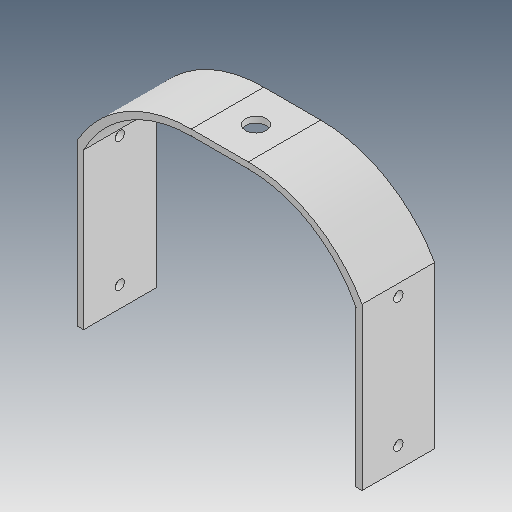
# Autodesk Inventor part: shin_bracket
Saved by Autodesk Inventor 2025.2 (Build 292293000, 293)
## iProperties
Created: 2025-02-16
Part Number: shin_bracket
Material: Generic
Document SubType Name: Modeling
Designer: email
Density: 1 g/cm^3
Appearance: Default
Author: email
Autodesk Inventor part; units mm, degrees
ref_plane "YZ Plane" through (0, 0, 0) normal (1, 0, 0) x (0, 1, 0)
ref_plane "XZ Plane" through (0, 0, 0) normal (0, 1, 0) x (-1, 0, 0)
ref_plane "XY Plane" through (0, 0, 0) normal (0, 0, 1) x (1, 0, 0)
sketch "Sketch1" plane through (0, 0, 0) normal (0, 0, 1) x (1, 0, 0)
  line L0 (0, 0) -> (3.2, 0)
  line L1 (3.2, 0) -> (3.2, 82)
  line L2 (0, 0) -> (0, 85)
  line L3 (146.8, 82) -> (146.8, 0)
  line L4 (146.8, 0) -> (150, 0)
  line L5 (150, 0) -> (150, 85)
  arc A0 (60, 116.8) -> (3.2, 82) centre (60, 53.046) ccw
  line L6 (60, 116.8) -> (90, 116.8)
  arc A1 (146.8, 82) -> (90, 116.8) centre (90, 53.046) ccw
  arc A2 (60, 120) -> (0, 85) centre (60, 51.0714) ccw
  line L7 (60, 120) -> (90, 120)
  arc A3 (150, 85) -> (90, 120) centre (90, 51.0714) ccw
  point P0 (75, 120)
  point P1 (75, 116.8)
  dimension "d0" = 3.2
  dimension "d1" = 3.2
  dimension "d2" = 3.2
  dimension "d3" = 150
  dimension "d4" = 120
  dimension "d5" = 30
  dimension "d12" = 85
  dimension "d13" = 75
  dimension "d14" = 3
  dimension "d15" = 30
  dimension "d16" = 85
  dimension "d17" = 8
  constraints: 16 end point, 8 point on circle, 4 centre point, 4 tangent, 3 perpendicular, 2 horizontal, 2 midpoint, 2 vertical, 1 collinear, 1 horizontal alignment, 1 parallel, 1 vertical alignment
  measures "d0" distance between parallel lines of L2 L1
  measures "d1" distance between parallel lines of L5 L3
  measures "d2" distance between parallel lines of L6 L7
  measures "d3" distance between parallel lines of L5 L2
  measures "d4" distance between parallel lines of L0 L7
  measures "d5" distance of L7.start L7.end
  measures "d12" distance of L4.end L5.end
  measures "d13" distance from line of L5 point (75, 120)
  measures "d14" vertical distance of L5.end L3.start
  measures "d15" distance of L6.start L6.end
  measures "d16" distance of L0.start L2.end
extrude "Extrusion1" add sketch "Sketch1" along normal blind 38.2
sketch "Sketch2" plane through (150, 0, 0) normal (1, 0, 0) x (0, 0, -1)
  circle A0 centre (-19.1, 11) radius 2.5
  circle A1 centre (-19.1, 79) radius 2.5
  line L0 (0, 0) -> (0, 85) projected
  line L1 (0, 0) -> (-38.2, 0) projected
  dimension "d8" = 19.1
  dimension "d9" = 5
  dimension "d10" = 68
  dimension "d11" = 11
  constraints: 2 centre point, 1 equal radius, 1 vertical alignment
  measures "d8" distance from line of L0 A1.centre
  measures "d9" diameter of A1
  measures "d10" distance of A0.centre A1.centre
  measures "d11" distance from line of L1 A0.centre
extrude "Extrusion2" cut sketch "Sketch2" against normal through all
sketch "Sketch3" plane through (60, 120, 0) normal (0, 1, 0) x (1, 0, 0)
  circle A0 centre (15, -19.1) radius 5.5
  line L0 (-60, 0) -> (-60, -38.2) projected
  line L1 (30, 0) -> (0, 0) projected
  dimension "d20" = 11
  dimension "d21" = 75
  dimension "d22" = 19.1
  constraints: 1 centre point
  measures "d20" diameter of A0
  measures "d21" distance from line of L0 A0.centre
  measures "d22" distance from line of L1 A0.centre
extrude "Extrusion3" cut sketch "Sketch3" against normal blind 10
body "Solid1"
